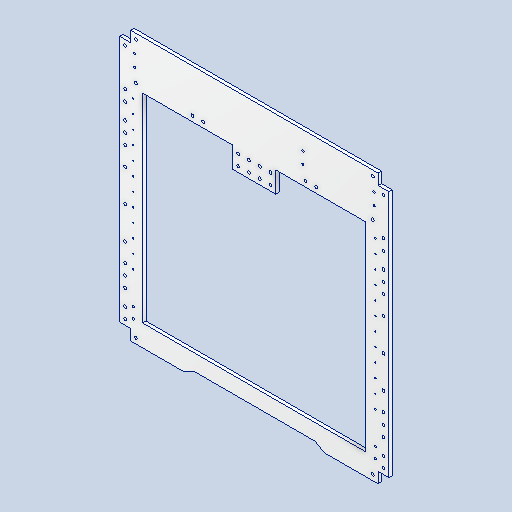
# Autodesk Inventor part: Printer Gantry Plate RevI
Saved by Autodesk Inventor 2024 (Build 280153000, 153)
## iProperties
Created: 2024-08-01
Part Number: Printer Gantry Plate RevI
Material: Aluminum 6061
Document SubType Name: Modeling
Designer: Ishaan
Density: 2.7 g/cm^3
Appearance: Aluminum - Flat
Author: Ishaan
Autodesk Inventor part; units mm, degrees
ref_plane "YZ Plane" through (0, 0, 0) normal (1, 0, 0) x (0, 1, 0)
ref_plane "XZ Plane" through (0, 0, 0) normal (0, 1, 0) x (-1, 0, 0)
ref_plane "XY Plane" through (0, 0, 0) normal (0, 0, 1) x (1, 0, 0)
sketch "Sketch1" plane through (0, 0, 0) normal (0, 0, 1) x (1, 0, 0)
  line L0 (253.25, -253.25) -> (-253.25, -253.25)
  line L1 (-253.25, -253.25) -> (-253.25, 253.25)
  line L2 (-253.25, 253.25) -> (253.25, 253.25)
  line L3 (253.25, 253.25) -> (253.25, -253.25)
  line L4 (253.25, -253.25) -> (-253.25, 253.25) construction
  line L5 (-253.25, -253.25) -> (253.25, 253.25) construction
  line L6 (-253.25, -253.25) -> (-233.25, -253.25) construction
  line L7 (-233.25, -253.25) -> (-233.25, -233.25) construction
  line L8 (-233.25, -233.25) -> (-253.25, -233.25) construction
  line L9 (-253.25, -233.25) -> (-253.25, -253.25) construction
  line L10 (-210, -250) -> (-250, -250) construction
  line L11 (-250, -250) -> (-250, -210) construction
  line L12 (-250, -210) -> (-210, -210) construction
  line L13 (-210, -210) -> (-210, -250) construction
  line L14 (-210, -250) -> (-250, -210) construction
  line L15 (-250, -250) -> (-210, -210) construction
  line L16 (-220, -240) -> (-240, -240) construction
  line L17 (-240, -240) -> (-240, -220) construction
  line L18 (-240, -220) -> (-220, -220) construction
  line L19 (-220, -220) -> (-220, -240) construction
  line L20 (-220, -240) -> (-240, -220) construction
  line L21 (-240, -240) -> (-220, -220) construction
  line L22 (253.25, -253.25) -> (233.25, -253.25) construction
  line L23 (233.25, -253.25) -> (233.25, -233.25) construction
  line L24 (233.25, -233.25) -> (253.25, -233.25) construction
  line L25 (253.25, -233.25) -> (253.25, -253.25) construction
  line L26 (210, -210) -> (250, -210) construction
  line L27 (250, -210) -> (250, -250) construction
  line L28 (250, -250) -> (210, -250) construction
  line L29 (210, -250) -> (210, -210) construction
  line L30 (210, -210) -> (250, -250) construction
  line L31 (250, -210) -> (210, -250) construction
  line L32 (240, -240) -> (220, -240) construction
  line L33 (220, -240) -> (220, -220) construction
  line L34 (220, -220) -> (240, -220) construction
  line L35 (240, -220) -> (240, -240) construction
  line L36 (240, -240) -> (220, -220) construction
  line L37 (220, -240) -> (240, -220) construction
  line L38 (-253.25, 253.25) -> (-233.25, 253.25) construction
  line L39 (-233.25, 253.25) -> (-233.25, 233.25) construction
  line L40 (-233.25, 233.25) -> (-253.25, 233.25) construction
  line L41 (-253.25, 233.25) -> (-253.25, 253.25) construction
  line L42 (253.25, 253.25) -> (233.25, 253.25) construction
  line L43 (233.25, 253.25) -> (233.25, 233.25) construction
  line L44 (233.25, 233.25) -> (253.25, 233.25) construction
  line L45 (253.25, 233.25) -> (253.25, 253.25) construction
  line L46 (210, 210) -> (250, 210) construction
  line L47 (250, 210) -> (250, 250) construction
  line L48 (250, 250) -> (210, 250) construction
  line L49 (210, 250) -> (210, 210) construction
  line L50 (210, 210) -> (250, 250) construction
  line L51 (250, 210) -> (210, 250) construction
  line L52 (240, 220) -> (220, 220) construction
  line L53 (220, 220) -> (220, 240) construction
  line L54 (220, 240) -> (240, 240) construction
  line L55 (240, 240) -> (240, 220) construction
  line L56 (240, 220) -> (220, 240) construction
  line L57 (220, 220) -> (240, 240) construction
  line L58 (-210, 210) -> (-250, 210) construction
  line L59 (-250, 210) -> (-250, 250) construction
  line L60 (-250, 250) -> (-210, 250) construction
  line L61 (-210, 250) -> (-210, 210) construction
  line L62 (-210, 210) -> (-250, 250) construction
  line L63 (-250, 210) -> (-210, 250) construction
  line L64 (-240, 220) -> (-220, 220) construction
  line L65 (-220, 220) -> (-220, 240) construction
  line L66 (-220, 240) -> (-240, 240) construction
  line L67 (-240, 240) -> (-240, 220) construction
  line L68 (-240, 220) -> (-220, 240) construction
  line L69 (-220, 220) -> (-240, 240) construction
  line L70 (250, 140) -> (210, 140) construction
  line L71 (210, 140) -> (210, 180) construction
  line L72 (210, 180) -> (250, 180) construction
  line L73 (250, 180) -> (250, 140) construction
  line L74 (250, 140) -> (210, 180) construction
  line L75 (210, 140) -> (250, 180) construction
  line L76 (240, 150) -> (220, 150) construction
  line L77 (220, 150) -> (220, 170) construction
  line L78 (220, 170) -> (240, 170) construction
  line L79 (240, 170) -> (240, 150) construction
  line L80 (240, 150) -> (220, 170) construction
  line L81 (220, 150) -> (240, 170) construction
  line L82 (-40, 161) -> (40, 161) construction
  line L83 (40, 161) -> (40, 121) construction
  line L84 (40, 121) -> (-40, 121) construction
  line L85 (-40, 121) -> (-40, 161) construction
  line L86 (-40, 161) -> (40, 121) construction
  line L87 (40, 161) -> (-40, 121) construction
  line L88 (30, 131) -> (-30, 131) construction
  line L89 (-30, 131) -> (-30, 151) construction
  line L90 (-30, 151) -> (30, 151) construction
  line L91 (30, 151) -> (30, 131) construction
  line L92 (30, 131) -> (-30, 151) construction
  line L93 (-30, 131) -> (30, 151) construction
  line L94 (10, 131) -> (-10, 131) construction
  line L95 (-10, 131) -> (-10, 151) construction
  line L96 (-10, 151) -> (10, 151) construction
  line L97 (10, 151) -> (10, 131) construction
  line L98 (10, 131) -> (-10, 151) construction
  line L99 (-10, 131) -> (10, 151) construction
  line L100 (125, 160) -> (85, 160) construction
  line L101 (85, 160) -> (85, 180) construction
  line L102 (85, 180) -> (125, 180) construction
  line L103 (125, 180) -> (125, 160) construction
  line L104 (125, 160) -> (85, 180) construction
  line L105 (85, 160) -> (125, 180) construction
  line L106 (95, 170) -> (115, 170) construction
  line L107 (-210, 140) -> (-250, 140) construction
  line L108 (-250, 140) -> (-250, 180) construction
  line L109 (-250, 180) -> (-210, 180) construction
  line L110 (-210, 180) -> (-210, 140) construction
  line L111 (-210, 140) -> (-250, 180) construction
  line L112 (-250, 140) -> (-210, 180) construction
  line L113 (-240, 150) -> (-220, 150) construction
  line L114 (-220, 150) -> (-220, 170) construction
  line L115 (-220, 170) -> (-240, 170) construction
  line L116 (-240, 170) -> (-240, 150) construction
  line L117 (-240, 150) -> (-220, 170) construction
  line L118 (-220, 150) -> (-240, 170) construction
  line L119 (-85, 160) -> (-125, 160) construction
  line L120 (-125, 160) -> (-125, 180) construction
  line L121 (-125, 180) -> (-85, 180) construction
  line L122 (-85, 180) -> (-85, 160) construction
  line L123 (-85, 160) -> (-125, 180) construction
  line L124 (-125, 160) -> (-85, 180) construction
  line L125 (-115, 170) -> (-95, 170) construction
  line L126 (-230, 50) -> (-250, 50) construction
  line L127 (-250, 50) -> (-250, 90) construction
  line L128 (-250, 90) -> (-230, 90) construction
  line L129 (-230, 90) -> (-230, 50) construction
  line L130 (-230, 50) -> (-250, 90) construction
  line L131 (-250, 50) -> (-230, 90) construction
  line L132 (-240, 60) -> (-240, 80) construction
  line L133 (250, 50) -> (230, 50) construction
  line L134 (230, 50) -> (230, 90) construction
  line L135 (230, 90) -> (250, 90) construction
  line L136 (250, 90) -> (250, 50) construction
  line L137 (250, 50) -> (230, 90) construction
  line L138 (230, 50) -> (250, 90) construction
  line L139 (240, 80) -> (240, 60) construction
  line L140 (-253.25, -233.25) -> (-233.25, -253.25) construction
  line L141 (253.25, -233.25) -> (233.25, -253.25) construction
  line L142 (233.25, 253.25) -> (253.25, 233.25) construction
  line L143 (-253.25, 233.25) -> (-233.25, 253.25) construction
  line L144 (253.25, -253.25) -> (250, -253.25)
  line L145 (250, -253.25) -> (250, 250)
  line L146 (250, 250) -> (253.25, 250)
  line L147 (253.25, 250) -> (253.25, -253.25)
  line L148 (253.25, 250) -> (-253.25, 250)
  line L149 (-253.25, 250) -> (-253.25, 253.25)
  line L150 (-253.25, 253.25) -> (253.25, 253.25)
  line L151 (253.25, 253.25) -> (253.25, 250)
  line L152 (-253.25, 250) -> (-250, 250)
  line L153 (-250, 250) -> (-250, -250)
  line L154 (-250, -250) -> (-253.25, -250)
  line L155 (-253.25, -250) -> (-253.25, 250)
  line L156 (-253.25, -253.25) -> (250, -253.25)
  line L157 (250, -253.25) -> (250, -250)
  line L158 (250, -250) -> (-253.25, -250)
  line L159 (-253.25, -250) -> (-253.25, -253.25)
  line L160 (-230, -160) -> (-250, -160) construction
  line L161 (-250, -160) -> (-250, -120) construction
  line L162 (-250, -120) -> (-230, -120) construction
  line L163 (-230, -120) -> (-230, -160) construction
  line L164 (-230, -160) -> (-250, -120) construction
  line L165 (-250, -160) -> (-230, -120) construction
  line L166 (-240, -130) -> (-240, -150) construction
  line L167 (250, -160) -> (230, -160) construction
  line L168 (230, -160) -> (230, -120) construction
  line L169 (230, -120) -> (250, -120) construction
  line L170 (250, -120) -> (250, -160) construction
  line L171 (250, -160) -> (230, -120) construction
  line L172 (230, -160) -> (250, -120) construction
  line L173 (240, -150) -> (240, -130) construction
  point P0 (0, 0)
  point P1 (-230, -230)
  point P2 (230, -230)
  point P3 (230, 230)
  point P4 (-230, 230)
  point P5 (230, 160)
  point P6 (0, 141)
  point P7 (85, 170)
  point P8 (105, 170)
  point P9 (-230, 160)
  point P10 (-105, 170)
  point P11 (-240, 70)
  point P12 (240, 70)
  point P13 (-243.25, 243.25)
  point P14 (243.25, 243.25)
  point P15 (243.25, -243.25)
  point P16 (-243.25, -243.25)
  point P17 (-250, -250)
  point P18 (250, -250)
  point P19 (250, 250)
  point P20 (-240, -140)
  point P21 (240, -140)
  dimension "d0" = 506.5
  dimension "d1" = 506.5
  dimension "d2" = 20
  dimension "d3" = 20
  dimension "d4" = 40
  dimension "d5" = 40
  dimension "d6" = 3.25
  dimension "d7" = 3.25
  dimension "d8" = 20
  dimension "d9" = 20
  dimension "d10" = 3.25
  dimension "d11" = 3.25
  dimension "d12" = 3.25
  dimension "d13" = 3.25
  dimension "d14" = 3.25
  dimension "d15" = 3.25
  dimension "d16" = 3.25
  dimension "d17" = 70
  dimension "d18" = 80
  dimension "d19" = 40
  dimension "d20" = 60
  dimension "d21" = 20
  dimension "d22" = 20
  dimension "d23" = 20
  dimension "d24" = 40
  dimension "d25" = 20
  dimension "d27" = 85
  dimension "d28" = 20
  dimension "d30" = 20
  dimension "d113" = 85
  dimension "d115" = 50
  dimension "d136" = 1
  dimension "d137" = 50
  dimension "d138" = 50
  dimension "d139" = 50
  dimension "d140" = 170
  dimension "d141" = 170
  constraints: 348 end point, 60 parallel, 55 midpoint, 40 equal length, 32 coincident, 32 horizontal, 30 perpendicular, 6 collinear, 4 vertical, 3 vertical alignment
  measures "d0" distance of L1.end L2.end
  measures "d1" distance of L0.end L1.end
  measures "d2" distance of L8.end L7.end
  measures "d3" distance of L7.end L6.end
  measures "d4" distance of L11.end L12.end
  measures "d5" distance of L10.end L11.end
  measures "d6" distance between parallel lines of L11 L1
  measures "d7" distance between parallel lines of L0 L10
  measures "d8" distance of L17.end L18.end
  measures "d9" distance of L16.end L17.end
  measures "d10" distance between parallel lines of L0 L28
  measures "d11" distance between parallel lines of L3 L27
  measures "d12" distance between parallel lines of L2 L48
  measures "d13" distance between parallel lines of L3 L47
  measures "d14" distance between parallel lines of L2 L60
  measures "d15" distance between parallel lines of L59 L1
  measures "d16" distance between parallel lines of L3 L73
  measures "d17" distance between parallel lines of L72 L48
  measures "d18" distance of L83.end L84.end
  measures "d19" distance of L82.end L83.end
  measures "d20" distance of L89.end L90.end
  measures "d21" distance of L88.end L89.end
  measures "d22" distance of L95.end L96.end
  measures "d23" distance of L94.end L95.end
  measures "d24" distance of L101.end L102.end
  measures "d25" distance of L100.end L101.end
  measures "d27" distance between parallel lines of L103 L71
  measures "d28" distance of L106.start L106.end
  measures "d30" distance of L125.start L125.end
  measures "d113" distance between parallel lines of L120 L110
  measures "d115" distance between parallel lines of L128 L107
  measures "d136" distance between parallel lines of L82 L100
  measures "d137" distance between parallel lines of L12 L160
  measures "d138" distance between parallel lines of L26 L167
  measures "d139" distance between parallel lines of L135 L70
  measures "d140" distance between parallel lines of L162 L126
  measures "d141" distance between parallel lines of L101 L122
extrude "Extrusion1" add sketch "Sketch1" along normal blind 6.35 contours L158 L153 L148 L145
hole "Hole1" at (-240, -220, 0) at (-220, -240, 0) at (220, -240, 0) at (240, -220, 0) at (220, 240, 0) at (240, 220, 0) at (-240, 220, 0) at (-220, 240, 0) at (220, 170, 0) at (240, 150, 0) at (-30, 151, 0) at (-30, 131, 0) at (-10, 151, 0) at (-10, 131, 0) at (10, 151, 0) at (10, 131, 0) at (30, 151, 0) at (30, 131, 0) at (95, 170, 0) at (115, 170, 0) at (-220, 170, 0) at (-240, 150, 0) at (-115, 170, 0) at (-95, 170, 0) at (-240, 80, 0) at (-240, 60, 0) at (240, 80, 0) at (240, 60, 0) at (-243.25, 243.25, 0) at (243.25, 243.25, 0) at (243.25, -243.25, 0) at (-243.25, -243.25, 0) at (-240, -130, 0) at (-240, -150, 0) at (240, -130, 0) at (240, -150, 0) direction (0, 0, 1) diameter 5.3 end through all
sketch "Sketch2" plane through (0, 0, 6.35) normal (0, 0, 1) x (1, 0, 0)
  circle A0 centre (-243.25, -243.25) radius 2.65 projected
  circle A1 centre (243.25, -243.25) radius 2.65 projected
  circle A2 centre (243.25, 243.25) radius 2.65 projected
  circle A3 centre (-243.25, 243.25) radius 2.65 projected
  circle A4 centre (240, 60) radius 2.65 projected
  circle A5 centre (240, 80) radius 2.65 projected
  circle A6 centre (-240, 60) radius 2.65 projected
  circle A7 centre (-240, 80) radius 2.65 projected
  circle A8 centre (-95, 170) radius 2.65 projected
  circle A9 centre (-115, 170) radius 2.65 projected
  circle A10 centre (-240, 150) radius 2.65 projected
  circle A11 centre (-220, 170) radius 2.65 projected
  circle A12 centre (115, 170) radius 2.65 projected
  circle A13 centre (95, 170) radius 2.65 projected
  circle A14 centre (30, 131) radius 2.65 projected
  circle A15 centre (30, 151) radius 2.65 projected
  circle A16 centre (10, 131) radius 2.65 projected
  circle A17 centre (10, 151) radius 2.65 projected
  circle A18 centre (-10, 131) radius 2.65 projected
  circle A19 centre (-10, 151) radius 2.65 projected
  circle A20 centre (-30, 131) radius 2.65 projected
  circle A21 centre (-30, 151) radius 2.65 projected
  circle A22 centre (240, 150) radius 2.65 projected
  circle A23 centre (220, 170) radius 2.65 projected
  circle A24 centre (-220, 240) radius 2.65 projected
  circle A25 centre (-240, 220) radius 2.65 projected
  circle A26 centre (240, 220) radius 2.65 projected
  circle A27 centre (220, 240) radius 2.65 projected
  circle A28 centre (240, -220) radius 2.65 projected
  circle A29 centre (220, -240) radius 2.65 projected
  circle A30 centre (-220, -240) radius 2.65 projected
  circle A31 centre (-240, -220) radius 2.65 projected
  line L0 (-250, 250) -> (-230, 250)
  line L1 (-230, 250) -> (-230, 230)
  line L2 (-230, 230) -> (-250, 230)
  line L3 (-250, 230) -> (-250, 250)
  line L4 (250, 250) -> (230, 250)
  line L5 (230, 250) -> (230, 230)
  line L6 (230, 230) -> (250, 230)
  line L7 (250, 230) -> (250, 250)
  line L8 (250, -250) -> (230, -250)
  line L9 (230, -250) -> (230, -230)
  line L10 (230, -230) -> (250, -230)
  line L11 (250, -230) -> (250, -250)
  line L12 (-250, -250) -> (-230, -250)
  line L13 (-230, -250) -> (-230, -230)
  line L14 (-230, -230) -> (-250, -230)
  line L15 (-250, -230) -> (-250, -250)
  point P0 (0, 0)
  dimension "d43" = 20
  dimension "d44" = 20
  constraints: 32 end point, 8 parallel, 6 equal length, 4 coincident, 4 horizontal, 4 perpendicular
  measures "d43" distance of L1.end L2.end
  measures "d44" distance of L0.end L1.end
extrude "Extrusion2" cut sketch "Sketch2" against normal through all contours A0 | L0 L1 L2 L3 | L7 L6 L5 L4 | L8 L9 L10 L11 | L15 L14 L13 L12
sketch "Sketch4" plane through (0, 0, 6.35) normal (0, 0, 1) x (1, 0, 0)
  line L0 (230, -250) -> (230, -230) projected
  line L1 (230, -230) -> (250, -230) projected
  line L2 (250, -230) -> (250, 230) projected
  line L3 (250, 230) -> (230, 230) projected
  line L4 (230, 230) -> (230, 250) projected
  line L5 (230, 250) -> (-230, 250) projected
  line L6 (-230, 250) -> (-230, 230) projected
  line L7 (-230, 230) -> (-250, 230) projected
  line L8 (-250, 230) -> (-250, -230) projected
  line L9 (-250, -230) -> (-230, -230) projected
  line L10 (-230, -230) -> (-230, -250) projected
  line L11 (-230, -250) -> (230, -250) projected
  circle A0 centre (-240, -220) radius 2.65 projected
  circle A1 centre (-220, -240) radius 2.65 projected
  circle A2 centre (220, -240) radius 2.65 projected
  circle A3 centre (240, -220) radius 2.65 projected
  circle A4 centre (220, 240) radius 2.65 projected
  circle A5 centre (240, 220) radius 2.65 projected
  circle A6 centre (-240, 220) radius 2.65 projected
  circle A7 centre (-220, 240) radius 2.65 projected
  circle A8 centre (220, 170) radius 2.65 projected
  circle A9 centre (240, 150) radius 2.65 projected
  circle A10 centre (-30, 151) radius 2.65 projected
  circle A11 centre (-30, 131) radius 2.65 projected
  circle A12 centre (-10, 151) radius 2.65 projected
  circle A13 centre (-10, 131) radius 2.65 projected
  circle A14 centre (10, 151) radius 2.65 projected
  circle A15 centre (10, 131) radius 2.65 projected
  circle A16 centre (30, 151) radius 2.65 projected
  circle A17 centre (30, 131) radius 2.65 projected
  circle A18 centre (95, 170) radius 2.65 projected
  circle A19 centre (115, 170) radius 2.65 projected
  circle A20 centre (-220, 170) radius 2.65 projected
  circle A21 centre (-240, 150) radius 2.65 projected
  circle A22 centre (-115, 170) radius 2.65 projected
  circle A23 centre (-95, 170) radius 2.65 projected
  circle A24 centre (-240, 80) radius 2.65 projected
  circle A25 centre (-240, 60) radius 2.65 projected
  circle A26 centre (240, 80) radius 2.65 projected
  circle A27 centre (240, 60) radius 2.65 projected
  line L12 (-250, -250) -> (-210, -250) construction
  line L13 (-210, -250) -> (-210, -210) construction
  line L14 (-210, -210) -> (-250, -210) construction
  line L15 (-250, -210) -> (-250, -250) construction
  line L16 (250, -250) -> (210, -250) construction
  line L17 (210, -250) -> (210, -210) construction
  line L18 (210, -210) -> (250, -210) construction
  line L19 (250, -210) -> (250, -250) construction
  line L20 (-210, -250) -> (-130, -250)
  line L21 (-130, -250) -> (-112.6795, -240)
  line L22 (-112.6795, -240) -> (112.6795, -240)
  line L23 (112.6795, -240) -> (130, -250)
  line L24 (210, -250) -> (130, -250)
  line L25 (210, -214) -> (-210, -214)
  line L26 (-210, -214) -> (-210, -250)
  line L27 (210, -214) -> (210, -250)
  line L28 (-207.5, -210) -> (207.5, -210)
  line L29 (207.5, -210) -> (207.5, 121)
  line L30 (207.5, 121) -> (-207.5, 121)
  line L31 (-207.5, 121) -> (-207.5, -210)
  line L32 (-10, 151) -> (10, 131) construction
  line L33 (40, 121) -> (-40, 121) construction
  line L34 (-40, 121) -> (-40, 161) construction
  line L35 (-40, 161) -> (40, 161) construction
  line L36 (40, 161) -> (40, 121) construction
  line L37 (40, 121) -> (-40, 161) construction
  line L38 (-40, 121) -> (40, 161) construction
  line L39 (-240, 150) -> (-220, 170) construction
  line L40 (220, 170) -> (240, 150) construction
  line L41 (250, 140) -> (210, 140) construction
  line L42 (210, 140) -> (210, 180) construction
  line L43 (210, 180) -> (250, 180) construction
  line L44 (250, 180) -> (250, 140) construction
  line L45 (250, 140) -> (210, 180) construction
  line L46 (210, 140) -> (250, 180) construction
  line L47 (-210, 140) -> (-250, 140) construction
  line L48 (-250, 140) -> (-250, 180) construction
  line L49 (-250, 180) -> (-210, 180) construction
  line L50 (-210, 180) -> (-210, 140) construction
  line L51 (-210, 140) -> (-250, 180) construction
  line L52 (-250, 140) -> (-210, 180) construction
  line L53 (-115, 170) -> (-95, 170) construction
  line L54 (95, 170) -> (115, 170) construction
  line L55 (125, 160) -> (85, 160) construction
  line L56 (85, 160) -> (85, 180) construction
  line L57 (85, 180) -> (125, 180) construction
  line L58 (125, 180) -> (125, 160) construction
  line L59 (125, 160) -> (85, 180) construction
  line L60 (85, 160) -> (125, 180) construction
  line L61 (-85, 160) -> (-125, 160) construction
  line L62 (-125, 160) -> (-125, 180) construction
  line L63 (-125, 180) -> (-85, 180) construction
  line L64 (-85, 180) -> (-85, 160) construction
  line L65 (-85, 160) -> (-125, 180) construction
  line L66 (-125, 160) -> (-85, 180) construction
  line L67 (-210, 160) -> (-40, 160)
  line L68 (-40, 160) -> (-40, 121)
  line L69 (-40, 121) -> (-210, 121)
  line L70 (-210, 121) -> (-210, 160)
  line L71 (40, 160) -> (210, 160)
  line L72 (210, 160) -> (210, 140)
  line L73 (210, 140) -> (40, 140)
  line L74 (40, 140) -> (40, 160)
  line L75 (-207.5, 121) -> (-210, 121)
  line L76 (-210, 121) -> (-210, 160)
  line L77 (-210, 160) -> (-207.5, 160)
  line L78 (-207.5, 160) -> (-207.5, 121)
  line L79 (207.5, 121) -> (210, 121)
  line L80 (210, 121) -> (210, 160)
  line L81 (210, 160) -> (207.5, 160)
  line L82 (207.5, 160) -> (207.5, 121)
  line L83 (-210, 160) -> (-125, 160)
  line L84 (-125, 160) -> (-125, 176)
  line L85 (-125, 176) -> (-210, 176)
  line L86 (-210, 176) -> (-210, 160)
  line L87 (-85, 160) -> (-40, 160)
  line L88 (-40, 160) -> (-40, 176)
  line L89 (-40, 176) -> (-85, 176)
  line L90 (-85, 176) -> (-85, 160)
  line L91 (40, 160) -> (85, 160)
  line L92 (85, 160) -> (85, 176)
  line L93 (85, 176) -> (40, 176)
  line L94 (40, 176) -> (40, 160)
  line L95 (125, 160) -> (210, 160)
  line L96 (210, 160) -> (210, 176)
  line L97 (210, 176) -> (125, 176)
  line L98 (125, 176) -> (125, 160)
  line L99 (-210, -210) -> (210, -210)
  line L100 (210, -210) -> (210, -214)
  line L101 (210, -214) -> (-210, -214)
  line L102 (-210, -214) -> (-210, -210)
  line L103 (40, 140) -> (40, 121)
  point P0 (0, 0)
  point P1 (0, -240)
  point P2 (0, 141)
  point P3 (230, 160)
  point P4 (-230, 160)
  point P5 (105, 170)
  point P6 (-105, 170)
  point P7 (-190, -190)
  point P8 (190, -190)
  point P9 (210, 140)
  point P10 (-210, 118)
  point P11 (125, 160)
  point P12 (85, 160)
  point P13 (-85, 160)
  point P14 (-125, 160)
  point P15 (210, -210)
  point P16 (40, 121)
  point P17 (210, 118)
  point P18 (0, -210)
  point P19 (-207.5, 160)
  point P20 (207.5, 160)
  dimension "d67" = 40
  dimension "d68" = 40
  dimension "d70" = 80
  dimension "d71" = 80
  dimension "d72" = 10
  dimension "d73" = 150
  dimension "d81" = 80
  dimension "d82" = 40
  dimension "d83" = 40
  dimension "d84" = 40
  dimension "d85" = 40
  dimension "d86" = 40
  dimension "d87" = 40
  dimension "d88" = 20
  dimension "d89" = 40
  dimension "d90" = 20
  dimension "d93" = 4
  dimension "d94" = 4
  dimension "d132" = 415
  constraints: 184 end point, 36 parallel, 20 perpendicular, 19 horizontal, 18 midpoint, 14 point on line, 11 collinear, 2 vertical alignment
  measures "d67" distance of L16.end L17.end
  measures "d68" distance between parallel lines of L19 L17
  measures "d70" distance from line of L13 L20.end
  measures "d71" distance from line of L17 L23.end
  measures "d72" distance between parallel lines of L22 L11
  measures "d73" angle of L11 L23
  measures "d81" distance of L34.end L35.end
  measures "d82" distance of L33.end L34.end
  measures "d83" distance of L42.end L43.end
  measures "d84" distance of L41.end L42.end
  measures "d85" distance of L48.end L49.end
  measures "d86" distance of L47.end L48.end
  measures "d87" distance of L56.end L57.end
  measures "d88" distance of L55.end L56.end
  measures "d89" distance of L62.end L63.end
  measures "d90" distance of L61.end L62.end
  measures "d93" distance between parallel lines of L63 L85
  measures "d94" distance between parallel lines of L25 L28
  measures "d132" distance between parallel lines of L29 L31
extrude "Extrusion3" cut sketch "Sketch4" against normal through all contours L11 L21 L22 L23
extrude "Extrusion4" cut sketch "Sketch4" against normal through all contours L28 L31 L30 L29 | L30 L103 L73 L82 | L78 L67 L68 L30 | L73 L74 L71 L82
sketch "Sketch5" plane through (0, 0, 6.35) normal (0, 0, 1) x (1, 0, 0)
  line L0 (207.5, -210) -> (-207.5, -210) projected
  line L1 (-207.5, 160) -> (-40, 160) projected
  line L2 (-40, 160) -> (-40, 121) projected
  line L3 (-40, 121) -> (40, 121) projected
  line L4 (40, 121) -> (40, 160) projected
  line L5 (112.6795, -240) -> (130, -250) projected
  line L6 (130, -250) -> (230, -250) projected
  line L7 (230, -250) -> (230, -230) projected
  line L8 (230, -230) -> (250, -230) projected
  line L9 (250, -230) -> (250, 230) projected
  line L10 (250, 230) -> (230, 230) projected
  line L11 (230, 230) -> (230, 250) projected
  line L12 (230, 250) -> (-230, 250) projected
  line L13 (-230, 250) -> (-230, 230) projected
  line L14 (-230, 230) -> (-250, 230) projected
  line L15 (-250, 230) -> (-250, -230) projected
  line L16 (-250, -230) -> (-230, -230) projected
  line L17 (-230, -230) -> (-230, -250) projected
  line L18 (-230, -250) -> (-130, -250) projected
  line L19 (-130, -250) -> (-112.6795, -240) projected
  line L20 (-112.6795, -240) -> (112.6795, -240) projected
  circle A0 centre (-240, -220) radius 2.65 projected
  circle A1 centre (-220, -240) radius 2.65 projected
  circle A2 centre (220, -240) radius 2.65 projected
  circle A3 centre (240, -220) radius 2.65 projected
  circle A4 centre (220, 240) radius 2.65 projected
  circle A5 centre (240, 220) radius 2.65 projected
  circle A6 centre (-240, 220) radius 2.65 projected
  circle A7 centre (-220, 240) radius 2.65 projected
  circle A8 centre (220, 170) radius 2.65 projected
  circle A9 centre (240, 150) radius 2.65 projected
  circle A10 centre (-30, 151) radius 2.65 projected
  circle A11 centre (-30, 131) radius 2.65 projected
  circle A12 centre (-10, 151) radius 2.65 projected
  circle A13 centre (-10, 131) radius 2.65 projected
  circle A14 centre (10, 151) radius 2.65 projected
  circle A15 centre (10, 131) radius 2.65 projected
  circle A16 centre (30, 151) radius 2.65 projected
  circle A17 centre (30, 131) radius 2.65 projected
  circle A18 centre (95, 170) radius 2.65 projected
  circle A19 centre (115, 170) radius 2.65 projected
  circle A20 centre (-220, 170) radius 2.65 projected
  circle A21 centre (-240, 150) radius 2.65 projected
  circle A22 centre (-115, 170) radius 2.65 projected
  circle A23 centre (-95, 170) radius 2.65 projected
  circle A24 centre (-240, 80) radius 2.65 projected
  circle A25 centre (-240, 60) radius 2.65 projected
  circle A26 centre (240, 80) radius 2.65 projected
  circle A27 centre (240, 60) radius 2.65 projected
  line L21 (-225, -132.5) -> (-225, 142.5) construction
  line L22 (-219, -145) -> (-231, -145) construction
  line L23 (-231, -145) -> (-231, 155) construction
  line L24 (-231, 155) -> (-219, 155) construction
  line L25 (-219, 155) -> (-219, -145) construction
  line L26 (-219, -145) -> (-231, 155) construction
  line L27 (-231, -145) -> (-219, 155) construction
  line L28 (40, 160) -> (207.5, 160) projected
  line L29 (207.5, 160) -> (207.5, -210) projected
  line L30 (-207.5, -210) -> (-207.5, 160) projected
  point P0 (0, 0)
  point P1 (-225, -107.5)
  point P2 (-225, -82.5)
  point P3 (-225, -57.5)
  point P4 (-225, -32.5)
  point P5 (-225, -7.5)
  point P6 (-225, 17.5)
  point P7 (-225, 42.5)
  point P8 (-225, 67.5)
  point P9 (-225, 92.5)
  point P10 (-225, 117.5)
  point P11 (-225, 5)
  dimension "d97" = 25
  dimension "d102" = 12
  dimension "d103" = 300
  dimension "d104" = 25
  dimension "d105" = 95
  constraints: 14 end point, 3 midpoint, 2 parallel, 2 vertical, 1 horizontal, 1 perpendicular, 11 other
  measures "d97" distance of L21.start point (-225, -107.5)
  measures "d102" distance of L23.end L24.end
  measures "d103" distance of L22.end L23.end
  measures "d104" distance from line of point (-225, 42.5) L15
  measures "d105" distance between parallel lines of L12 L24
hole "Hole2" at (-225, -132.5, 6.35) at (-225, -107.5, 6.35) at (-225, -82.5, 6.35) at (-225, -57.5, 6.35) at (-225, -32.5, 6.35) at (-225, -7.5, 6.35) at (-225, 17.5, 6.35) at (-225, 42.5, 6.35) at (-225, 67.5, 6.35) at (-225, 92.5, 6.35) at (-225, 117.5, 6.35) at (-225, 142.5, 6.35) direction (0, 0, -1) diameter 2.459 end through all thread size "M3x0.5" class "6H" standard "ANSI Metric M Profile"
mirror "Mirror1" about plane through (0, 0, 0) normal (1, 0, 0) of "Hole2"
sketch "Sketch6" plane through (0, 0, 6.35) normal (0, 0, 1) x (1, 0, 0)
  circle A0 centre (225, 142.5) radius 1.2295 projected
  circle A1 centre (225, -132.5) radius 1.2295 projected
  circle A2 centre (225, -107.5) radius 1.2295 projected
  circle A3 centre (225, -82.5) radius 1.2295 projected
  circle A4 centre (225, -57.5) radius 1.2295 projected
  circle A5 centre (225, -32.5) radius 1.2295 projected
  circle A6 centre (225, -7.5) radius 1.2295 projected
  circle A7 centre (225, 17.5) radius 1.2295 projected
  circle A8 centre (225, 42.5) radius 1.2295 projected
  circle A9 centre (225, 67.5) radius 1.2295 projected
  circle A10 centre (225, 92.5) radius 1.2295 projected
  circle A11 centre (225, 117.5) radius 1.2295 projected
  circle A12 centre (-225, 142.5) radius 1.2295 projected
  circle A13 centre (-225, 117.5) radius 1.2295 projected
  circle A14 centre (-225, 92.5) radius 1.2295 projected
  circle A15 centre (-225, 67.5) radius 1.2295 projected
  circle A16 centre (-225, 42.5) radius 1.2295 projected
  circle A17 centre (-225, 17.5) radius 1.2295 projected
  circle A18 centre (-225, -7.5) radius 1.2295 projected
  circle A19 centre (-225, -32.5) radius 1.2295 projected
  circle A20 centre (-225, -57.5) radius 1.2295 projected
  circle A21 centre (-225, -82.5) radius 1.2295 projected
  circle A22 centre (-225, -107.5) radius 1.2295 projected
  circle A23 centre (-225, -132.5) radius 1.2295 projected
  line L0 (207.5, -210) -> (-207.5, -210) projected
  line L1 (-207.5, 160) -> (-40, 160) projected
  line L2 (-40, 160) -> (-40, 121) projected
  line L3 (-40, 121) -> (40, 121) projected
  line L4 (40, 121) -> (40, 160) projected
  line L5 (112.6795, -240) -> (130, -250) projected
  line L6 (130, -250) -> (230, -250) projected
  line L7 (230, -250) -> (230, -230) projected
  line L8 (230, -230) -> (250, -230) projected
  line L9 (250, -230) -> (250, 230) projected
  line L10 (250, 230) -> (230, 230) projected
  line L11 (230, 230) -> (230, 250) projected
  line L12 (230, 250) -> (-230, 250) projected
  line L13 (-230, 250) -> (-230, 230) projected
  line L14 (-230, 230) -> (-250, 230) projected
  line L15 (-250, 230) -> (-250, -230) projected
  line L16 (-250, -230) -> (-230, -230) projected
  line L17 (-230, -230) -> (-230, -250) projected
  line L18 (-230, -250) -> (-130, -250) projected
  line L19 (-130, -250) -> (-112.6795, -240) projected
  line L20 (-112.6795, -240) -> (112.6795, -240) projected
  circle A24 centre (240, 60) radius 2.65 projected
  circle A25 centre (240, 80) radius 2.65 projected
  circle A26 centre (-240, 60) radius 2.65 projected
  circle A27 centre (-240, 80) radius 2.65 projected
  circle A28 centre (-95, 170) radius 2.65 projected
  circle A29 centre (-115, 170) radius 2.65 projected
  circle A30 centre (-240, 150) radius 2.65 projected
  circle A31 centre (-220, 170) radius 2.65 projected
  circle A32 centre (115, 170) radius 2.65 projected
  circle A33 centre (95, 170) radius 2.65 projected
  circle A34 centre (30, 131) radius 2.65 projected
  circle A35 centre (30, 151) radius 2.65 projected
  circle A36 centre (10, 131) radius 2.65 projected
  circle A37 centre (10, 151) radius 2.65 projected
  circle A38 centre (-10, 131) radius 2.65 projected
  circle A39 centre (-10, 151) radius 2.65 projected
  circle A40 centre (-30, 131) radius 2.65 projected
  circle A41 centre (-30, 151) radius 2.65 projected
  circle A42 centre (240, 150) radius 2.65 projected
  circle A43 centre (220, 170) radius 2.65 projected
  circle A44 centre (-220, 240) radius 2.65 projected
  circle A45 centre (-240, 220) radius 2.65 projected
  circle A46 centre (240, 220) radius 2.65 projected
  circle A47 centre (220, 240) radius 2.65 projected
  circle A48 centre (240, -220) radius 2.65 projected
  circle A49 centre (220, -240) radius 2.65 projected
  circle A50 centre (-220, -240) radius 2.65 projected
  circle A51 centre (-240, -220) radius 2.65 projected
  line L21 (222.5, 194) -> (-222.5, 194) construction
  line L22 (-222.5, 194) -> (-222.5, 216) construction
  line L23 (-222.5, 216) -> (222.5, 216) construction
  line L24 (222.5, 216) -> (222.5, 194) construction
  line L25 (222.5, 194) -> (-222.5, 216) construction
  line L26 (-222.5, 194) -> (222.5, 216) construction
  line L27 (90.5, 216) -> (90.5, 194) construction
  line L28 (40, 160) -> (207.5, 160) projected
  line L29 (207.5, 160) -> (207.5, -210) projected
  line L30 (-207.5, -210) -> (-207.5, 160) projected
  line L31 (225, -212) -> (-225, -212) construction
  line L32 (-225, -212) -> (-225, -192) construction
  line L33 (-225, -192) -> (225, -192) construction
  line L34 (225, -192) -> (225, -212) construction
  line L35 (225, -212) -> (-225, -192) construction
  line L36 (-225, -212) -> (225, -192) construction
  point P0 (0, 0)
  point P1 (0, 205)
  point P2 (0, -202)
  dimension "d120" = 22
  dimension "d121" = 34
  dimension "d122" = 27.5
  dimension "d131" = 132
  dimension "d133" = 20
  dimension "d134" = 25
  dimension "d135" = 18
  constraints: 26 end point, 10 coincident, 4 midpoint, 4 parallel, 3 perpendicular, 2 horizontal, 2 point on line, 2 vertical alignment
  measures "d120" distance of L21.end L22.end
  measures "d121" distance between parallel lines of L23 L12
  measures "d122" distance between parallel lines of L22 L15
  measures "d131" distance between parallel lines of L27 L24
  measures "d133" distance of L31.end L32.end
  measures "d134" distance between parallel lines of L32 L15
  measures "d135" distance between parallel lines of L31 L16
hole "Hole3" at (222.5, 216, 6.35) at (222.5, 194, 6.35) at (-222.5, 216, 6.35) at (-222.5, 194, 6.35) at (90.5, 216, 6.35) at (90.5, 194, 6.35) at (225, -192, 6.35) at (225, -212, 6.35) at (-225, -192, 6.35) at (-225, -212, 6.35) direction (0, 0, -1) diameter 4.134 end through all thread size "M5x0.8" class "6H" standard "ANSI Metric M Profile"
sketch "Sketch7" plane through (0, 0, 6.35) normal (0, 0, 1) x (1, 0, 0)
  circle A0 centre (-225, -212) radius 2.067 projected
  circle A1 centre (-225, -192) radius 2.067 projected
  circle A2 centre (225, -212) radius 2.067 projected
  circle A3 centre (225, -192) radius 2.067 projected
  circle A4 centre (90.5, 194) radius 2.067 projected
  circle A5 centre (90.5, 216) radius 2.067 projected
  circle A6 centre (-222.5, 194) radius 2.067 projected
  circle A7 centre (-222.5, 216) radius 2.067 projected
  circle A8 centre (222.5, 194) radius 2.067 projected
  circle A9 centre (222.5, 216) radius 2.067 projected
  circle A10 centre (225, 142.5) radius 1.2295 projected
  circle A11 centre (225, -132.5) radius 1.2295 projected
  circle A12 centre (225, -107.5) radius 1.2295 projected
  circle A13 centre (225, -82.5) radius 1.2295 projected
  circle A14 centre (225, -57.5) radius 1.2295 projected
  circle A15 centre (225, -32.5) radius 1.2295 projected
  circle A16 centre (225, -7.5) radius 1.2295 projected
  circle A17 centre (225, 17.5) radius 1.2295 projected
  circle A18 centre (225, 42.5) radius 1.2295 projected
  circle A19 centre (225, 67.5) radius 1.2295 projected
  circle A20 centre (225, 92.5) radius 1.2295 projected
  circle A21 centre (225, 117.5) radius 1.2295 projected
  circle A22 centre (-225, 142.5) radius 1.2295 projected
  circle A23 centre (-225, 117.5) radius 1.2295 projected
  circle A24 centre (-225, 92.5) radius 1.2295 projected
  circle A25 centre (-225, 67.5) radius 1.2295 projected
  circle A26 centre (-225, 42.5) radius 1.2295 projected
  circle A27 centre (-225, 17.5) radius 1.2295 projected
  circle A28 centre (-225, -7.5) radius 1.2295 projected
  circle A29 centre (-225, -32.5) radius 1.2295 projected
  circle A30 centre (-225, -57.5) radius 1.2295 projected
  circle A31 centre (-225, -82.5) radius 1.2295 projected
  circle A32 centre (-225, -107.5) radius 1.2295 projected
  circle A33 centre (-225, -132.5) radius 1.2295 projected
  line L0 (40, 160) -> (207.5, 160) projected
  line L1 (207.5, 160) -> (207.5, -210) projected
  line L2 (207.5, -210) -> (-207.5, -210) projected
  line L3 (-207.5, -210) -> (-207.5, 160) projected
  line L4 (-207.5, 160) -> (-40, 160) projected
  line L5 (-40, 160) -> (-40, 121) projected
  line L6 (-40, 121) -> (40, 121) projected
  line L7 (40, 121) -> (40, 160) projected
  line L8 (112.6795, -240) -> (130, -250) projected
  line L9 (130, -250) -> (230, -250) projected
  line L10 (230, -250) -> (230, -230) projected
  line L11 (230, -230) -> (250, -230) projected
  line L12 (250, -230) -> (250, 230) projected
  line L13 (250, 230) -> (230, 230) projected
  line L14 (230, 230) -> (230, 250) projected
  line L15 (230, 250) -> (-230, 250) projected
  line L16 (-230, 250) -> (-230, 230) projected
  line L17 (-230, 230) -> (-250, 230) projected
  line L18 (-250, 230) -> (-250, -230) projected
  line L19 (-250, -230) -> (-230, -230) projected
  line L20 (-230, -230) -> (-230, -250) projected
  line L21 (-230, -250) -> (-130, -250) projected
  line L22 (-130, -250) -> (-112.6795, -240) projected
  line L23 (-112.6795, -240) -> (112.6795, -240) projected
  circle A34 centre (240, -150) radius 2.65 projected
  circle A35 centre (240, -130) radius 2.65 projected
  circle A36 centre (-240, -150) radius 2.65 projected
  circle A37 centre (-240, -130) radius 2.65 projected
  circle A38 centre (240, 60) radius 2.65 projected
  circle A39 centre (240, 80) radius 2.65 projected
  circle A40 centre (-240, 60) radius 2.65 projected
  circle A41 centre (-240, 80) radius 2.65 projected
  circle A42 centre (-95, 170) radius 2.65 projected
  circle A43 centre (-115, 170) radius 2.65 projected
  circle A44 centre (-240, 150) radius 2.65 projected
  circle A45 centre (-220, 170) radius 2.65 projected
  circle A46 centre (115, 170) radius 2.65 projected
  circle A47 centre (95, 170) radius 2.65 projected
  circle A48 centre (30, 131) radius 2.65 projected
  circle A49 centre (30, 151) radius 2.65 projected
  circle A50 centre (10, 131) radius 2.65 projected
  circle A51 centre (10, 151) radius 2.65 projected
  circle A52 centre (-10, 131) radius 2.65 projected
  circle A53 centre (-10, 151) radius 2.65 projected
  circle A54 centre (-30, 131) radius 2.65 projected
  circle A55 centre (-30, 151) radius 2.65 projected
  circle A56 centre (240, 150) radius 2.65 projected
  circle A57 centre (220, 170) radius 2.65 projected
  circle A58 centre (-220, 240) radius 2.65 projected
  circle A59 centre (-240, 220) radius 2.65 projected
  circle A60 centre (240, 220) radius 2.65 projected
  circle A61 centre (220, 240) radius 2.65 projected
  circle A62 centre (240, -220) radius 2.65 projected
  circle A63 centre (220, -240) radius 2.65 projected
  circle A64 centre (-220, -240) radius 2.65 projected
  circle A65 centre (-240, -220) radius 2.65 projected
  line L24 (240, 150) -> (240, 80) construction
  line L25 (240, 130) -> (240, 100) construction
  line L26 (240, -150) -> (240, -220) construction
  line L27 (240, -170) -> (240, -200) construction
  line L28 (-240, 150) -> (-240, 80) construction
  line L29 (-240, 130) -> (-240, 100) construction
  line L30 (-240, -150) -> (-240, -220) construction
  line L31 (-240, -170) -> (-240, -200) construction
  point P0 (0, 0)
  point P1 (240, 115)
  point P2 (240, -185)
  point P3 (-240, 115)
  point P4 (-240, -185)
  dimension "d142" = 30
  dimension "d143" = 30
  dimension "d144" = 30
  dimension "d145" = 30
  constraints: 16 end point, 10 coincident, 8 midpoint, 7 vertical, 1 perpendicular
  measures "d142" distance of L25.start L25.end
  measures "d143" distance of L27.start L27.end
  measures "d144" distance of L29.start L29.end
  measures "d145" distance of L31.start L31.end
hole "Hole4" at (240, 130, 6.35) at (240, 100, 6.35) at (240, -170, 6.35) at (240, -200, 6.35) at (-240, 130, 6.35) at (-240, 100, 6.35) at (-240, -170, 6.35) at (-240, -200, 6.35) direction (0, 0, -1) diameter 5.4 end through all
sketch "Sketch8" plane through (0, 0, 6.35) normal (0, 0, 1) x (1, 0, 0)
  circle A0 centre (-240, -200) radius 2.7 projected
  circle A1 centre (-240, -170) radius 2.7 projected
  circle A2 centre (-240, 100) radius 2.7 projected
  circle A3 centre (-240, 130) radius 2.7 projected
  circle A4 centre (240, -200) radius 2.7 projected
  circle A5 centre (240, -170) radius 2.7 projected
  circle A6 centre (240, 100) radius 2.7 projected
  circle A7 centre (240, 130) radius 2.7 projected
  circle A8 centre (-225, -212) radius 2.067 projected
  circle A9 centre (-225, -192) radius 2.067 projected
  circle A10 centre (225, -212) radius 2.067 projected
  circle A11 centre (225, -192) radius 2.067 projected
  circle A12 centre (90.5, 194) radius 2.067 projected
  circle A13 centre (90.5, 216) radius 2.067 projected
  circle A14 centre (-222.5, 194) radius 2.067 projected
  circle A15 centre (-222.5, 216) radius 2.067 projected
  circle A16 centre (222.5, 194) radius 2.067 projected
  circle A17 centre (222.5, 216) radius 2.067 projected
  circle A18 centre (225, 142.5) radius 1.2295 projected
  circle A19 centre (225, -132.5) radius 1.2295 projected
  circle A20 centre (225, -107.5) radius 1.2295 projected
  circle A21 centre (225, -82.5) radius 1.2295 projected
  circle A22 centre (225, -57.5) radius 1.2295 projected
  circle A23 centre (225, -32.5) radius 1.2295 projected
  circle A24 centre (225, -7.5) radius 1.2295 projected
  circle A25 centre (225, 17.5) radius 1.2295 projected
  circle A26 centre (225, 42.5) radius 1.2295 projected
  circle A27 centre (225, 67.5) radius 1.2295 projected
  circle A28 centre (225, 92.5) radius 1.2295 projected
  circle A29 centre (225, 117.5) radius 1.2295 projected
  circle A30 centre (-225, 142.5) radius 1.2295 projected
  circle A31 centre (-225, 117.5) radius 1.2295 projected
  circle A32 centre (-225, 92.5) radius 1.2295 projected
  circle A33 centre (-225, 67.5) radius 1.2295 projected
  circle A34 centre (-225, 42.5) radius 1.2295 projected
  circle A35 centre (-225, 17.5) radius 1.2295 projected
  circle A36 centre (-225, -7.5) radius 1.2295 projected
  circle A37 centre (-225, -32.5) radius 1.2295 projected
  circle A38 centre (-225, -57.5) radius 1.2295 projected
  circle A39 centre (-225, -82.5) radius 1.2295 projected
  circle A40 centre (-225, -107.5) radius 1.2295 projected
  circle A41 centre (-225, -132.5) radius 1.2295 projected
  line L0 (40, 160) -> (207.5, 160) projected
  line L1 (207.5, 160) -> (207.5, -210) projected
  line L2 (207.5, -210) -> (-207.5, -210) projected
  line L3 (-207.5, -210) -> (-207.5, 160) projected
  line L4 (-207.5, 160) -> (-40, 160) projected
  line L5 (-40, 160) -> (-40, 121) projected
  line L6 (-40, 121) -> (40, 121) projected
  line L7 (40, 121) -> (40, 160) projected
  line L8 (112.6795, -240) -> (130, -250) projected
  line L9 (130, -250) -> (230, -250) projected
  line L10 (230, -250) -> (230, -230) projected
  line L11 (230, -230) -> (250, -230) projected
  line L12 (250, -230) -> (250, 230) projected
  line L13 (250, 230) -> (230, 230) projected
  line L14 (230, 230) -> (230, 250) projected
  line L15 (230, 250) -> (-230, 250) projected
  line L16 (-230, 250) -> (-230, 230) projected
  line L17 (-230, 230) -> (-250, 230) projected
  line L18 (-250, 230) -> (-250, -230) projected
  line L19 (-250, -230) -> (-230, -230) projected
  line L20 (-230, -230) -> (-230, -250) projected
  line L21 (-230, -250) -> (-130, -250) projected
  line L22 (-130, -250) -> (-112.6795, -240) projected
  line L23 (-112.6795, -240) -> (112.6795, -240) projected
  circle A42 centre (240, -150) radius 2.65 projected
  circle A43 centre (240, -130) radius 2.65 projected
  circle A44 centre (-240, -150) radius 2.65 projected
  circle A45 centre (-240, -130) radius 2.65 projected
  circle A46 centre (240, 60) radius 2.65 projected
  circle A47 centre (240, 80) radius 2.65 projected
  circle A48 centre (-240, 60) radius 2.65 projected
  circle A49 centre (-240, 80) radius 2.65 projected
  circle A50 centre (-95, 170) radius 2.65 projected
  circle A51 centre (-115, 170) radius 2.65 projected
  circle A52 centre (-240, 150) radius 2.65 projected
  circle A53 centre (-220, 170) radius 2.65 projected
  circle A54 centre (115, 170) radius 2.65 projected
  circle A55 centre (95, 170) radius 2.65 projected
  circle A56 centre (30, 131) radius 2.65 projected
  circle A57 centre (30, 151) radius 2.65 projected
  circle A58 centre (10, 131) radius 2.65 projected
  circle A59 centre (10, 151) radius 2.65 projected
  circle A60 centre (-10, 131) radius 2.65 projected
  circle A61 centre (-10, 151) radius 2.65 projected
  circle A62 centre (-30, 131) radius 2.65 projected
  circle A63 centre (-30, 151) radius 2.65 projected
  circle A64 centre (240, 150) radius 2.65 projected
  circle A65 centre (220, 170) radius 2.65 projected
  circle A66 centre (-220, 240) radius 2.65 projected
  circle A67 centre (-240, 220) radius 2.65 projected
  circle A68 centre (240, 220) radius 2.65 projected
  circle A69 centre (220, 240) radius 2.65 projected
  circle A70 centre (240, -220) radius 2.65 projected
  circle A71 centre (220, -240) radius 2.65 projected
  circle A72 centre (-220, -240) radius 2.65 projected
  circle A73 centre (-240, -220) radius 2.65 projected
  line L24 (240, 25) -> (240, -95) construction
  line L25 (240, 60) -> (240, -130) construction
  line L26 (-240, 60) -> (-240, -130) construction
  line L27 (-240, 25) -> (-240, -95) construction
  point P0 (0, 0)
  point P1 (-240, -35)
  point P2 (240, -35)
  dimension "d153" = 120
  dimension "d49" = 50
  dimension "d50" = 42
  dimension "d56" = 300
  dimension "d57" = 250
  dimension "d59" = 50
  dimension "d60" = 400
  dimension "d61" = 12
  dimension "d62" = 12
  dimension "d63" = 300
  dimension "d64" = 15
  dimension "d65" = 27
  dimension "d66" = 45
  constraints: 8 end point, 4 coincident, 4 midpoint, 4 vertical, 1 parallel
  measures "d153" distance of L24.start L24.end
hole "Hole5" at (240, 25, 6.35) at (240, -95, 6.35) at (-240, 25, 6.35) at (-240, -95, 6.35) at (-240, -35, 6.35) at (240, -35, 6.35) direction (0, 0, -1) diameter 5.4 end through all
equation "\"d10\" = d7"
equation "\"d11\" = d6"
equation "\"d12\" = d10"
equation "\"d13\" = d11"
equation "\"d14\" = d12"
equation "\"d15\" = d13"
equation "\"d16\" = d13"
equation "\"d68\" = d67"
equation "\"d71\" = d70"
equation "\"d93\" = d78"
equation "\"d78\" = 4"
body "Solid1"
